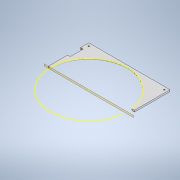
# Autodesk Inventor part: Drop_Plate
Saved by Autodesk Inventor 2022 (Build 260153000, 153)
## iProperties
Created: 2023-02-27
Part Number: Drop_Plate
Material: Generic
Document SubType Name: Modeling
Designer: zarek
Density: 1 g/cm^3
Appearance: Default
Author: zarek
Autodesk Inventor part; units mm, degrees
ref_plane "YZ Plane" through (0, 0, 0) normal (1, 0, 0) x (0, 1, 0)
ref_plane "XZ Plane" through (0, 0, 0) normal (0, 1, 0) x (-1, 0, 0)
ref_plane "XY Plane" through (0, 0, 0) normal (0, 0, 1) x (1, 0, 0)
sketch "Sketch1" plane through (0, 0, 0) normal (0, 1, 0) x (-1, 0, 0)
  line L0 (101.6, -101.6) -> (-101.6, -101.6)
  line L1 (-101.6, -101.6) -> (-101.6, 101.6)
  line L2 (-101.6, 101.6) -> (101.6, 101.6)
  line L3 (101.6, 101.6) -> (101.6, -101.6)
  line L4 (96.6, -96.6) -> (-96.6, -96.6)
  line L5 (-96.6, -96.6) -> (-96.6, 96.6)
  line L6 (-96.6, 96.6) -> (96.6, 96.6)
  line L7 (96.6, 96.6) -> (96.6, -96.6)
  line L8 (101.6, 101.6) -> (-40.4, 101.6)
  circle A0 centre (0, 0) radius 88.9
  line L9 (-40.4, 101.6) -> (-101.6, 40.4)
  line L10 (-45.4, 101.6) -> (-101.6, 45.4)
  line L11 (96.6, 96.6) -> (96.6, 101.6)
  line L12 (-45.4, 101.6) -> (-35.4, 101.6)
  line L13 (-35.4, 101.6) -> (-35.4, 96.6)
  line L14 (-35.4, 96.6) -> (-45.4, 96.6)
  line L15 (-45.4, 96.6) -> (-45.4, 101.6)
  line L16 (-101.6, 39.4) -> (-39.4, 101.6)
  line L17 (96.4, -96.4) -> (-96.4, -96.4)
  line L18 (-96.4, -96.4) -> (-96.4, 96.4)
  line L19 (-96.4, 96.4) -> (96.4, 96.4)
  line L20 (96.4, 96.4) -> (96.4, -96.4)
  circle A1 centre (0, 0) radius 90.9
  point P0 (96.6, 51.2168)
  point P1 (101.6, 40.4)
  point P2 (101.6, -40.4)
  point P3 (96.6, -51.2168)
  point P4 (-96.6, 45.4)
  point P5 (-45.4, 96.6)
  point P6 (-44.6, 96.4)
  point P7 (-96.4, 44.6)
  dimension "d0" = 203.2
  dimension "d1" = 203.2
  dimension "d2" = 101.6
  dimension "d3" = 101.6
  dimension "d4" = 5
  dimension "d5" = 5
  dimension "d6" = 5
  dimension "d7" = 5
  dimension "d8" = 142
  dimension "d9" = 61.2
  dimension "d10" = 177.8
  dimension "d11" = 5
  dimension "d12" = 5
  dimension "d13" = 10
  dimension "d14" = 1
  dimension "d15" = 0.2
  dimension "d16" = 0.2
  dimension "d17" = 0.2
  dimension "d18" = 0.2
  dimension "d64" = 181.8
  constraints: 42 end point, 10 parallel, 8 point on line, 5 perpendicular, 4 horizontal, 2 centre point, 2 coincident
  measures "d0" distance between parallel lines of L2 L0
  measures "d1" distance between parallel lines of L1 L3
  measures "d2" distance from line of L0 point (0, 0)
  measures "d3" distance from line of L1 point (0, 0)
  measures "d4" distance between parallel lines of L4 L0
  measures "d5" distance between parallel lines of L1 L5
  measures "d6" distance between parallel lines of L2 L6
  measures "d7" distance between parallel lines of L3 L7
  measures "d8" distance of L2.end L8.end
  measures "d9" distance from line of L1 L8.end
  measures "d10" diameter of A0
  measures "d11" distance of L10.end L9.end
  measures "d12" distance of L10.start L8.end
  measures "d13" distance of L13.end L14.end
  measures "d14" distance of L9.end L16.start
  measures "d15" distance between parallel lines of L5 L18
  measures "d16" distance between parallel lines of L4 L17
  measures "d17" distance between parallel lines of L7 L20
  measures "d18" distance between parallel lines of L6 L19
  measures "d64" diameter of A1
extrude "Extrusion1" add sketch "Sketch1" along normal blind 4 contours L16 L19 L20 L17 L18
sketch "Sketch6" plane through (0, 4, 0) normal (0, 1, 0) x (1, 0, 0)
  line L0 (96.4, 96.4) -> (-96.4, 96.4) projected
  line L1 (96.4, 96.4) -> (88.4, 96.4)
  line L2 (88.4, 96.4) -> (88.4, -45.6)
  line L3 (88.4, -45.6) -> (96.4, -45.6)
  line L4 (96.4, -45.6) -> (96.4, 96.4)
  line L5 (96.4, -44.6) -> (96.4, 96.4) projected
  line L6 (88.4, -12) -> (96.4, -12)
  line L7 (96.4, -12) -> (96.4, 12)
  line L8 (96.4, 12) -> (88.4, 12)
  line L9 (88.4, 12) -> (88.4, -12)
  line L10 (0, 0) -> (96.4, 0)
  point P0 (96.4, -12)
  dimension "d58" = 8
  dimension "d59" = 142
  dimension "d62" = 12
  dimension "d63" = 12
  constraints: 18 end point, 4 parallel, 3 perpendicular, 2 horizontal, 2 point on line, 1 midpoint
  measures "d58" distance of L3.end L2.end
  measures "d59" distance between parallel lines of L3 L0
  measures "d62" distance between parallel lines of L10 L8
  measures "d63" distance between parallel lines of L10 L6
extrude "Extrusion6" cut sketch "Sketch6" against normal blind 25.4 contours L4 L10 L2 L8 | L4 L6 L2 L10
sketch "Sketch8" plane through (0, 4, 0) normal (0, 1, 0) x (1, 0, 0)
  line L0 (-96.6, 96.6) -> (-96.6, -96.6)
  line L1 (96.6, 96.6) -> (-96.6, 96.6)
  line L2 (-96.6, 96.6) -> (96.6, 96.6)
  line L3 (96.6, -45.4) -> (45.4, -96.6)
  line L4 (96.6, 96.6) -> (96.6, -45.4)
  line L5 (96.6, -45.4) -> (45.4, -96.6)
  line L6 (45.4, -96.6) -> (-96.6, -96.6)
  line L7 (-96.6, -96.6) -> (-96.6, 96.6)
  line L8 (-96.6, 96.6) -> (-89.5289, 89.5289)
  circle A0 centre (-89.5289, 89.5289) radius 5
  circle A1 centre (-89.5289, 89.5289) radius 1.5
  line L9 (-89.5289, 84.5289) -> (-96.6, 84.5289)
  line L10 (-89.5289, 89.5289) -> (-89.5289, 84.5289)
  line L11 (-89.5289, 89.5289) -> (-84.5289, 89.5289)
  line L12 (-84.5289, 96.6) -> (-84.5289, 89.5289)
  line L13 (-96.6, -96.6) -> (-89.5289, -89.5289)
  line L14 (-96.6, -96.6) -> (-86.6, -96.6) construction
  circle A2 centre (-89.5289, -89.5289) radius 5
  circle A3 centre (-89.5289, -89.5289) radius 1.75
  line L15 (-89.5289, -89.5289) -> (-84.5289, -89.5289)
  line L16 (-84.5289, -96.6) -> (-84.5289, -89.5289)
  line L17 (-89.5289, -89.5289) -> (-89.5289, -84.5289)
  line L18 (-96.6, -84.5289) -> (-89.5289, -84.5289)
  line L19 (96.6, 96.6) -> (89.5289, 89.5289)
  circle A4 centre (89.5289, 89.5289) radius 5
  circle A5 centre (89.5289, 89.5289) radius 1.75
  line L20 (89.5289, 89.5289) -> (84.5289, 89.5289)
  line L21 (84.5289, 96.6) -> (84.5289, 89.5289)
  line L22 (89.5289, 89.5289) -> (89.5289, 84.5289)
  line L23 (96.6, 84.5289) -> (89.5289, 84.5289)
  line L24 (96.6, -43.114) -> (96.6, 96.6)
  line L25 (-96.6, -96.6) -> (43.1178, -96.6)
  line L26 (28.9914, 5.6569) -> (-5.6569, -28.9914)
  line L27 (25.4, -25.4) -> (101.6, -25.4)
  line L28 (101.6, -88.9) -> (101.6, 101.6)
  line L29 (25.4, -25.4) -> (25.4, -101.6)
  line L30 (43.1178, -101.6) -> (-101.6, -101.6)
  line L31 (96.6, -25.4) -> (86.6, -25.4)
  circle A6 centre (86.6, -25.4) radius 5
  circle A7 centre (86.6, -25.4) radius 1.75
  line L32 (25.4, -96.6) -> (25.4, -86.6)
  circle A8 centre (25.4, -86.6) radius 5
  circle A9 centre (25.4, -86.6) radius 1.75
  line L33 (44.6, -96.4) -> (96.4, -44.6) projected
  circle A10 centre (68.7322, -68.7322) radius 1
  point P0 (0, 0)
  point P1 (0, 0)
  point P2 (0, 0)
  dimension "d90" = 10
  dimension "d91" = 3
  dimension "d92" = 10
  dimension "d93" = 45
  dimension "d94" = 10
  dimension "d95" = 3.5
  dimension "d96" = 10
  dimension "d97" = 10
  dimension "d98" = 3.5
  dimension "d99" = 76.2
  dimension "d100" = 76.2
  dimension "d101" = 10
  dimension "d102" = 10
  dimension "d103" = 3.5
  dimension "d104" = 10
  dimension "d105" = 10
  dimension "d106" = 3.5
  dimension "d115" = 2
  dimension "d116" = 2.5
  constraints: 66 end point, 14 point on line, 11 centre point, 9 coincident, 9 perpendicular, 6 point on circle, 5 horizontal, 3 parallel, 2 tangent, 1 collinear, 1 equal length, 1 vertical
  measures "d90" distance of L0.start L8.end
  measures "d91" diameter of A1
  measures "d92" distance of L6.end L13.end
  measures "d93" angle of L14 L13
  measures "d94" diameter of A2
  measures "d95" diameter of A3
  measures "d96" distance of L1.start L19.end
  measures "d97" diameter of A4
  measures "d98" diameter of A5
  measures "d99" distance between parallel lines of L28 L29
  measures "d100" distance between parallel lines of L30 L27
  measures "d101" distance of L31.start L31.end
  measures "d102" diameter of A6
  measures "d103" diameter of A7
  measures "d104" distance of L32.start L32.end
  measures "d105" diameter of A8
  measures "d106" diameter of A9
  measures "d115" diameter of A10
  measures "d116" distance from line of L33 A10.centre
hole "Hole1" at (-89.5289, 4, -89.5289) at (89.5289, 4, -89.5289) at (-89.5289, 4, 89.5289) at (68.7322, 4, 68.7322) direction (0, -1, 0) diameter 3.1211 depth 2.75 tip angle 118 countersink diameter 3.2004 countersink angle 82 thread size "M3.5x0.35" class "6H" standard "ANSI Metric M Profile"
fillet "Fillet1" radius 3.175 2 edges at (-6.0132, 0, -90.7009) (-6.0132, 0, 90.7009)
sketch "Sketch9" plane through (0, 4, 0) normal (0, 1, 0) x (1, 0, 0)
  arc A0 (-101.6, -98.425) -> (-98.425, -101.6) centre (-98.425, -98.425) ccw
  line L0 (44.0849, 101.6) -> (-98.425, 101.6)
  line L1 (-101.6, 98.425) -> (-101.6, -98.425)
  line L2 (-101.6, -46.1) -> (-101.6, -76.6)
  line L3 (-96.6, -96.6) -> (-96.6, 96.6)
  line L4 (-96.6, -46.1) -> (-96.6, -76.6)
  line L5 (-101.6, -76.6) -> (-96.6, -76.6)
  line L6 (-101.6, -46.1) -> (-96.6, -46.1)
  line L7 (-98.425, -101.6) -> (101.6, -101.6)
  line L8 (0, 0) -> (-101.6, 0)
  line L9 (-101.6, 46.1) -> (-101.6, 76.6)
  line L10 (-96.6, 46.1) -> (-96.6, 76.6)
  line L11 (-101.6, 76.6) -> (-96.6, 76.6)
  line L12 (-101.6, 46.1) -> (-96.6, 46.1)
  line L13 (-96.6, -76.6) -> (-90.1, -76.6)
  line L14 (-90.1, -76.6) -> (-90.1, -46.1)
  line L15 (-90.1, -46.1) -> (-96.6, -46.1)
  line L16 (-96.6, -46.1) -> (-96.6, -76.6)
  arc A1 (-98.425, 101.6) -> (-101.6, 98.425) centre (-98.425, 98.425) ccw
  line L17 (-101.6, 46.1) -> (-96.6, 46.1)
  line L18 (-90.1, 46.1) -> (-96.6, 46.1)
  line L19 (-101.6, 46.1) -> (-101.6, 76.6)
  line L20 (-96.6, 46.1) -> (-96.6, 76.6)
  line L21 (-96.6, 46.1) -> (-96.6, 76.6)
  line L22 (-90.1, 76.6) -> (-90.1, 46.1)
  line L23 (-101.6, 76.6) -> (-96.6, 76.6)
  line L24 (-96.6, 76.6) -> (-90.1, 76.6)
  point P0 (-98.425, 98.425)
  point P1 (46.1, 101.6)
  point P2 (46.1, 96.6)
  point P3 (76.6, 96.6)
  point P4 (76.6, 101.6)
  point P5 (-46.1, 96.6)
  dimension "d117" = 30.5
  dimension "d118" = 25
  dimension "d119" = 6.5
  constraints: 50 end point, 10 symmetric about line, 4 point on circle, 3 parallel, 3 point on line, 2 centre point, 2 perpendicular, 1 horizontal, 1 midpoint, 1 other
  measures "d117" distance between parallel lines of L5 L6
  measures "d118" distance between parallel lines of L5 L7
  measures "d119" distance between parallel lines of L14 L3
extrude "Extrusion7" cut sketch "Sketch9" against normal blind 25.4 contours L24 L22 L18 L3 | L15 L14 L13 L3
sketch "Sketch10" plane through (0, 4, 0) normal (0, 1, 0) x (1, 0, 0)
  line L0 (-96.3514, 0) -> (-90.9, 0)
  arc A0 (90.1044, 12) -> (90.1044, -12) centre (0, 0) ccw projected
  constraints: 2 end point, 1 horizontal, 1 point on circle
ref_plane "Work Plane1" through (-96.3514, 4, 0) normal (0, 0, 1) x (1, 0, 0)
sketch "Sketch11" plane through (-96.3514, 4, 0) normal (0, 0, 1) x (1, 0, 0)
  line L0 (-51.1439, 37.1405) -> (237.6314, 37.1405)
  line L1 (237.6314, 37.1405) -> (237.6314, -59.6996)
  line L2 (237.6314, -59.6996) -> (-51.1439, -59.6996)
  line L3 (-51.1439, -59.6996) -> (-51.1439, 37.1405)
  point P0 (96.3514, -4)
  constraints: 8 end point, 2 parallel, 1 horizontal, 1 perpendicular
extrude "Extrusion8" cut sketch "Sketch11" along normal through all
equation "\"d1\" = d0"
equation "\"d2\" = 0.5 * d0"
equation "\"d3\" = 0.5 * d0"
equation "\"d15\" = d17"
equation "\"d16\" = d17"
equation "\"d18\" = d17"
body "Solid1"
